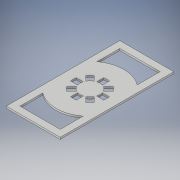
# Autodesk Inventor part: Cuerpo - Base
Saved by Autodesk Inventor 2019 (Build 230136000, 136)
## iProperties
Created: 2020-02-15
Part Number: Cuerpo - Base
Material: Genérico
Document SubType Name: Modeling
Designer: Mafer1
Density: 1 g/cm^3
Appearance: Valor por defecto
Mass: 62.4881 g
Surface Area: 432.904 cm^2
Volume: 62.4881 cm^3
ancho_base: 120.000 mm
largo_base: 200.000 mm
Author: Mafer1
Autodesk Inventor part; units mm, degrees
ref_plane "YZ Plane" through (0, 0, 0) normal (1, 0, 0) x (0, 1, 0)
ref_plane "XZ Plane" through (0, 0, 0) normal (0, 1, 0) x (-1, 0, 0)
ref_plane "XY Plane" through (0, 0, 0) normal (0, 0, 1) x (1, 0, 0)
sketch "Boceto1" plane through (0, 0, 0) normal (0, 1, 0) x (-1, 0, 0)
  line L0 (0, 0) -> (95, 0)
  line L1 (95, 0) -> (95, -200)
  line L2 (95, -200) -> (0, -200)
  line L3 (0, -200) -> (0, 0)
  dimension "d0" = 200
  dimension "d1" = 95
  constraints: 8 end point, 2 parallel, 1 horizontal, 1 perpendicular
  measures "d0" distance of L0.end L1.end
  measures "d1" distance between parallel lines of L3 L1
extrude "Extrusión1" add sketch "Boceto1" along normal blind 3.3
sketch "Boceto2" plane through (0, 3.3, 0) normal (0, 1, 0) x (1, 0, 0)
  circle A0 centre (-47.5, 100) radius 17.5 construction
  circle A1 centre (-47.5, 100) radius 29.5 construction
  line L0 (-83, 147.7493) -> (-83, 188)
  line L1 (-83, 188) -> (-12, 188)
  line L2 (-12, 188) -> (-12, 147.7493)
  line L3 (-83, 52.2507) -> (-83, 12)
  line L4 (-83, 12) -> (-12, 12)
  line L5 (-12, 12) -> (-12, 52.2507)
  arc A2 (-12, 147.7493) -> (-83, 147.7493) centre (-47.5, 100) ccw
  arc A3 (-83, 52.2507) -> (-12, 52.2507) centre (-47.5, 100) ccw
  line L6 (-95, 0) -> (0, 0) projected
  line L7 (0, 0) -> (0, 200) projected
  line L8 (0, 200) -> (-95, 200) projected
  line L9 (-95, 200) -> (-95, 0) projected
  line L10 (0, 200) -> (-95, 200) projected
  line L11 (-52.5, 70.9268) -> (-52.5, 83.2295)
  line L12 (-42.5, 70.9268) -> (-42.5, 83.2295)
  arc A4 (-52.5, 83.2295) -> (-42.5, 83.2295) centre (-47.5, 100) ccw
  arc A5 (-52.5, 70.9268) -> (-42.5, 70.9268) centre (-47.5, 100) ccw
  line L13 (-23.4066, 82.9777) -> (-32.1059, 91.677)
  arc A6 (-30.4777, 75.9066) -> (-23.4066, 82.9777) centre (-47.5, 100) ccw
  line L14 (-30.4777, 75.9066) -> (-39.177, 84.6059)
  arc A7 (-39.177, 84.6059) -> (-32.1059, 91.677) centre (-47.5, 100) ccw
  line L15 (-18.4268, 105) -> (-30.7295, 105)
  arc A8 (-18.4268, 95) -> (-18.4268, 105) centre (-47.5, 100) ccw
  line L16 (-18.4268, 95) -> (-30.7295, 95)
  arc A9 (-30.7295, 95) -> (-30.7295, 105) centre (-47.5, 100) ccw
  line L17 (-30.4777, 124.0934) -> (-39.177, 115.3941)
  arc A10 (-23.4066, 117.0223) -> (-30.4777, 124.0934) centre (-47.5, 100) ccw
  line L18 (-23.4066, 117.0223) -> (-32.1059, 108.323)
  arc A11 (-32.1059, 108.323) -> (-39.177, 115.3941) centre (-47.5, 100) ccw
  line L19 (-52.5, 129.0732) -> (-52.5, 116.7705)
  arc A12 (-42.5, 129.0732) -> (-52.5, 129.0732) centre (-47.5, 100) ccw
  line L20 (-42.5, 129.0732) -> (-42.5, 116.7705)
  arc A13 (-42.5, 116.7705) -> (-52.5, 116.7705) centre (-47.5, 100) ccw
  line L21 (-71.5934, 117.0223) -> (-62.8941, 108.323)
  arc A14 (-64.5223, 124.0934) -> (-71.5934, 117.0223) centre (-47.5, 100) ccw
  line L22 (-64.5223, 124.0934) -> (-55.823, 115.3941)
  arc A15 (-55.823, 115.3941) -> (-62.8941, 108.323) centre (-47.5, 100) ccw
  line L23 (-76.5732, 95) -> (-64.2705, 95)
  arc A16 (-76.5732, 105) -> (-76.5732, 95) centre (-47.5, 100) ccw
  line L24 (-76.5732, 105) -> (-64.2705, 105)
  arc A17 (-64.2705, 105) -> (-64.2705, 95) centre (-47.5, 100) ccw
  line L25 (-64.5223, 75.9066) -> (-55.823, 84.6059)
  arc A18 (-71.5934, 82.9777) -> (-64.5223, 75.9066) centre (-47.5, 100) ccw
  line L26 (-71.5934, 82.9777) -> (-62.8941, 91.677)
  arc A19 (-62.8941, 91.677) -> (-55.823, 84.6059) centre (-47.5, 100) ccw
  line L27 (-95, 200) -> (-95, 0) projected
  line L28 (0, 0) -> (0, 200) projected
  point P0 (-47.5, 200)
  point P1 (-95, 100)
  point P2 (-47.5, 200)
  point P3 (-47.5, 82.5)
  point P4 (-35.1256, 87.6256)
  point P5 (-30, 100)
  point P6 (-35.1256, 112.3744)
  point P7 (-47.5, 117.5)
  point P8 (-59.8744, 112.3744)
  point P9 (-65, 100)
  point P10 (-59.8744, 87.6256)
  dimension "d4" = 12
  dimension "d5" = 12
  dimension "d6" = 12
  dimension "d7" = 12
  dimension "d8" = 30
  dimension "d9" = 30
  dimension "d10" = 12
  dimension "d11" = 10
  dimension "d14" = 360
  dimension "d19" = 30
  constraints: 44 end point, 41 point on circle, 20 centre point, 4 concentric, 4 perpendicular, 3 midpoint, 3 parallel, 3 vertical, 3 vertical alignment, 2 point on line, 1 coincident, 1 collinear, 1 horizontal alignment, 89 other
  measures "d4" distance between parallel lines of L8 L1
  measures "d5" distance between parallel lines of L9 L0
  measures "d6" distance between parallel lines of L7 L2
  measures "d7" distance between parallel lines of L6 L4
  measures "d8" radial gap between concentric circles of A3 A1
  measures "d9" radial gap between concentric circles of A1 A2
  measures "d10" radial gap between concentric circles of A1 A0
  measures "d11" distance between parallel lines of L12 L11
  measures "d19" distance of point (-95, 100) point (-65, 100)
extrude "Extrusión2" cut sketch "Boceto2" against normal blind 10 contours L0 L1 L2 A2 | A3 L5 L4 L3 | L11 A4 L12 A5 | A6 L14 A7 L13 | A8 L16 A9 L15 | A10 L18 A11 L17 | A12 L20 A13 L19 | A14 L22 A15 L21 | A16 L24 A17 L23 | A18 L26 A19 L25
equation "\"d0\" = largo_base"
equation "\"d5\" = d4"
equation "\"d6\" = d4"
equation "\"d7\" = d4"
equation "\"d9\" = d8"
equation "\"d10\" = d4"
equation "\"d11\" = 0.333333 * d19"
equation "\"d19\" = d8"
equation "\"ancho_base\" = 120"
equation "\"largo_base\" = 200"
